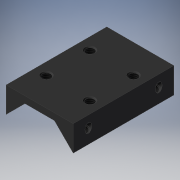
# Autodesk Inventor part: JKSGB10_b_b
Saved by Autodesk Inventor 2019 (Build 230136000, 136)
## iProperties
Created: 2024-06-28
Part Number: JKSGB10_b_b
Material: Generic
Catalog Web Link: www.cadenas.de
Description: JKSG, JKSC_block-Simplified Slide Guides for Jigs - Aluminum Bearing Type / Simplified Retention Type - Block Only
Vendor: MISUMI
Document SubType Name: Modeling
Designer: psAdmin
Manufacturer: MISUMI
Mass: 2.0327 g
Surface Area: 20.5359 cm^2
Volume: 2.0327 cm^3
Density: 1 g/cm^3
Appearance: PSOLRGB-175-175-175
Category: PARTsolutions
Company: MISUMI
Title: JKSGB10_b
Author: Cadenas PARTsolutions
Comments: Simplified Slide Guides for Jigs - Aluminum Bearing Type / Simplified Retention Type - Block Only
PSOL_IDENT_0: {$CADENAS_DATA/23d-libs/misumi/metric/07_slide_rails/jksgb.prj},172 {VTYP=3D},{NB=JKSGB10_b_b},{LINA=
PSOL_IDENT_1: JKSGB10_b},{NN=JKSG, JKSC_block},{DATE=30.06.2023 07:10:19},{GEOMDATE=09.06.2023 07:29:27},{VERSION=
PSOL_IDENT_2: },{LINEID=10},{WBVAR=TS},{WBNUMERIC=}  {NB=JKSGB10_b_b},{LINA=JKSGB10_b},{KT=DUMMY},{PN=JKSGB10_b},{
PSOL_IDENT_3: TS=SG},{TYPE=JKSG10},{MATB=Aluminum},{MATT=-},{MATTP=-},{STB=Hard Alumite Treatment},{H=10},{HALG=10
PSOL_IDENT_4: },{A=20},{B=30},{P1=13},{P2=13},{M=3},{MALG=[3]},{C=0.0},{D=0},{H1=7.5},{E=1.8},{F=7.6},{DGH=3.5x6x4
PSOL_IDENT_5: },{N=7.5},{P=40},{MB=F682ZZ},{SC=M2-5},{ALPB=49 (5)},{D1=2.000},{D4=10.000},{D6=10.500},{BD2=6.000},
PSOL_IDENT_6: {MMIN=1.567},{MMAX=2.000},{M1MIN=2.459},{M1MAX=3.000},{HT=10.000},{TTT=-0.100},{C2=0.600},{D2=3},{Q2=
PSOL_IDENT_7: 4.976},{TIF=1},{PPATH=jksgb_asmtpl.prj},{RF=0.0},{SH=3.6}
NB: JKSGB10_b_b
NN: JKSG, JKSC_block
NT: Simplified Slide Guides for Jigs - Aluminum Bearing Type / Simplified Retention Type - Block Only
NBSYN: $PN._b
LINA: JKSGB10_b
CATALOG: Misumi
PN: JKSGB10_b
TS: Aluminum Bearing
MATB: Aluminum
STB: Hard Alumite Treatment
HALG: 10
A: 20
B: 30
M: 3
ALPB: 49 (5)
PPATH: jksgb_asmtpl.prj
SUPPLIER: MISUMI
ARTICLENO: JKSGB10_b_b
BOMINFO: JKSGB10_b
CREATOR: CADENAS GmbH
Autodesk Inventor part; units mm, degrees
sketch "Sketch_1" plane through (0, 0, 0) normal (0, 0, 1) x (1, 0, 0)
  line L0 (-10, 2.4) -> (-4.4, 8)
  line L1 (-4.4, 8) -> (4.4, 8)
  line L2 (4.4, 8) -> (10, 2.4)
  line L3 (10, 2.4) -> (10, 10)
  line L4 (10, 10) -> (-10, 10)
  line L5 (-10, 10) -> (-10, 2.4)
  constraints: 12 end point
extrude "Extrusion1" add sketch "Sketch_1" along normal blind 30
sketch "Sketch_8" plane through (0, 0, 8.5) normal (0, 0, 1) x (1, 0, 0)
  line L0 (-6.5, 10) -> (-6.5, 4.4)
  line L1 (-6.5, 4.4) -> (-8, 4.4)
  line L2 (-8, 4.4) -> (-7.7295, 4.6705)
  line L3 (-7.7295, 4.6705) -> (-7.7295, 9.7295)
  line L4 (-7.7295, 9.7295) -> (-8, 10)
  line L5 (-8, 10) -> (-6.5, 10)
  line L6 (-6.5, 10) -> (-6.5, 4.4)
  constraints: 14 end point
revolve "Revolution1" cut sketch "Sketch_8" angle 360 about axis through (-6.5, 10, 8.5) along (0, 1, 0)
thread "Thread1" size "M3x0.5" class "6H" standard "ISO Metric profile" length 5.059
pattern_linear "Rectangular Pattern1" count 2 spacing 13 along (0, 0, 1) of "Revolution1"
sketch "Sketch_10" plane through (0, 0, 8.5) normal (0, 0, 1) x (1, 0, 0)
  line L0 (6.5, 4.4) -> (6.5, 10)
  line L1 (6.5, 10) -> (8, 10)
  line L2 (8, 10) -> (7.7295, 9.7295)
  line L3 (7.7295, 9.7295) -> (7.7295, 4.6705)
  line L4 (7.7295, 4.6705) -> (8, 4.4)
  line L5 (8, 4.4) -> (6.5, 4.4)
  line L6 (6.5, 4.4) -> (6.5, 10)
  constraints: 14 end point
revolve "Revolution2" cut sketch "Sketch_10" angle 360 about axis through (6.5, 4.4, 8.5) along (0, -1, 0)
thread "Thread2" size "M3x0.5" class "6H" standard "ISO Metric profile" length 5.059
pattern_linear "Rectangular Pattern2" count 2 spacing 13 along (0, 0, 1) of "Revolution2"
sketch "Sketch_2" plane through (0, 0, 25.5) normal (0, 0, 1) x (1, 0, 0)
  line L0 (-7.8787, 4.5213) -> (-10.7071, 7.3497)
  line L1 (-10.7071, 7.3497) -> (-10, 8.0569)
  line L2 (-10, 8.0569) -> (-8.5858, 6.6426)
  line L3 (-8.5858, 6.6426) -> (-8.5858, 6.3365)
  line L4 (-8.5858, 6.3365) -> (-7.4778, 5.2284)
  line L5 (-7.4778, 5.2284) -> (-7.1716, 5.2284)
  line L6 (-7.1716, 5.2284) -> (-7.8787, 4.5213)
  line L7 (-7.8787, 4.5213) -> (-10.7071, 7.3497)
  constraints: 16 end point
revolve "Revolution3" cut sketch "Sketch_2" angle 360 about axis through (-7.8787, 4.5213, 25.5) along (0.7071, -0.7071, 0)
thread "Thread3" size "M2x0.4" class "6H" standard "ISO Metric profile" full length
sketch "Sketch_4" plane through (0, 0, 25.5) normal (0, 0, 1) x (1, 0, 0)
  line L0 (10.7071, 7.3497) -> (7.8787, 4.5213)
  line L1 (7.8787, 4.5213) -> (7.1716, 5.2284)
  line L2 (7.1716, 5.2284) -> (7.4778, 5.2284)
  line L3 (7.4778, 5.2284) -> (8.5858, 6.3365)
  line L4 (8.5858, 6.3365) -> (8.5858, 6.6426)
  line L5 (8.5858, 6.6426) -> (10, 8.0569)
  line L6 (10, 8.0569) -> (10.7071, 7.3497)
  line L7 (10.7071, 7.3497) -> (7.8787, 4.5213)
  constraints: 16 end point
revolve "Revolution4" cut sketch "Sketch_4" angle 360 about axis through (10.7071, 7.3497, 25.5) along (0.7071, 0.7071, 0)
thread "Thread4" size "M2x0.4" class "6H" standard "ISO Metric profile" full length
sketch "Sketch_3" plane through (0, 0, 4.5) normal (0, 0, 1) x (1, 0, 0)
  line L0 (-7.8787, 4.5213) -> (-10.7071, 7.3497)
  line L1 (-10.7071, 7.3497) -> (-10, 8.0569)
  line L2 (-10, 8.0569) -> (-8.5858, 6.6426)
  line L3 (-8.5858, 6.6426) -> (-8.5858, 6.3365)
  line L4 (-8.5858, 6.3365) -> (-7.4778, 5.2284)
  line L5 (-7.4778, 5.2284) -> (-7.1716, 5.2284)
  line L6 (-7.1716, 5.2284) -> (-7.8787, 4.5213)
  line L7 (-7.8787, 4.5213) -> (-10.7071, 7.3497)
  constraints: 16 end point
revolve "Revolution5" cut sketch "Sketch_3" angle 360 about axis through (-7.8787, 4.5213, 4.5) along (0.7071, -0.7071, 0)
thread "Thread5" size "M2x0.4" class "6H" standard "ISO Metric profile" full length
sketch "Sketch_5" plane through (0, 0, 4.5) normal (0, 0, 1) x (1, 0, 0)
  line L0 (10.7071, 7.3497) -> (7.8787, 4.5213)
  line L1 (7.8787, 4.5213) -> (7.1716, 5.2284)
  line L2 (7.1716, 5.2284) -> (7.4778, 5.2284)
  line L3 (7.4778, 5.2284) -> (8.5858, 6.3365)
  line L4 (8.5858, 6.3365) -> (8.5858, 6.6426)
  line L5 (8.5858, 6.6426) -> (10, 8.0569)
  line L6 (10, 8.0569) -> (10.7071, 7.3497)
  line L7 (10.7071, 7.3497) -> (7.8787, 4.5213)
  constraints: 16 end point
revolve "Revolution6" cut sketch "Sketch_5" angle 360 about axis through (10.7071, 7.3497, 4.5) along (0.7071, 0.7071, 0)
thread "Thread6" size "M2x0.4" class "6H" standard "ISO Metric profile" full length
ref_plane "to_d_XY" through (0, 0, 15) normal (0, 0, 1) x (1, 0, 0)
ref_plane "to_d_YZ" through (0, 0, 15) normal (1, 0, 0) x (0, 1, 0)
ref_plane "to_d_ZX" through (0, 0, 15) normal (0, 1, 0) x (0, 0, 1)
ref_plane "to_rail_XY" through (0, 0, 15) normal (0, 0, 1) x (1, 0, 0)
ref_plane "to_rail_YZ" through (0, 0, 15) normal (1, 0, 0) x (0, 1, 0)
ref_plane "to_rail_ZX" through (0, 0, 15) normal (0, 1, 0) x (0, 0, 1)
ref_plane "to_sc1_XY" through (-7.8787, 4.5213, 4.5) normal (0.7071, -0.7071, 0) x (-0.7071, -0.7071, 0)
ref_plane "to_sc1_YZ" through (-7.8787, 4.5213, 4.5) normal (-0.7071, -0.7071, 0) x (0, 0, -1)
ref_plane "to_sc1_ZX" through (-7.8787, 4.5213, 4.5) normal (0, 0, -1) x (0.7071, -0.7071, 0)
ref_plane "to_sc12_XY" through (7.8787, 4.5213, 4.5) normal (0.7071, 0.7071, 0) x (0.7071, -0.7071, 0)
ref_plane "to_sc12_YZ" through (7.8787, 4.5213, 4.5) normal (0.7071, -0.7071, 0) x (0, 0, -1)
ref_plane "to_sc12_ZX" through (7.8787, 4.5213, 4.5) normal (0, 0, -1) x (0.7071, 0.7071, 0)
ref_plane "tosc2_XY" through (-7.8787, 4.5213, 25.5) normal (0.7071, -0.7071, 0) x (-0.7071, -0.7071, 0)
ref_plane "tosc2_YZ" through (-7.8787, 4.5213, 25.5) normal (-0.7071, -0.7071, 0) x (0, 0, -1)
ref_plane "tosc2_ZX" through (-7.8787, 4.5213, 25.5) normal (0, 0, -1) x (0.7071, -0.7071, 0)
ref_plane "tosc22_XY" through (7.8787, 4.5213, 25.5) normal (0.7071, 0.7071, 0) x (0.7071, -0.7071, 0)
ref_plane "tosc22_YZ" through (7.8787, 4.5213, 25.5) normal (0.7071, -0.7071, 0) x (0, 0, -1)
ref_plane "tosc22_ZX" through (7.8787, 4.5213, 25.5) normal (0, 0, -1) x (0.7071, 0.7071, 0)
body "Solid1"
